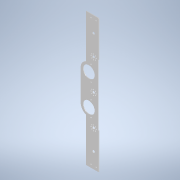
# Autodesk Inventor part: plate1
Saved by Autodesk Inventor 2020.1 (Build 241239000, 239)
## iProperties
Created: 2019-12-06
Part Number: plate1
Material: Aluminum 6061
Document SubType Name: Modeling
Designer: tbloo
Density: 2.7 g/cm^3
Appearance: Aluminum - Dark
Author: tbloo
Autodesk Inventor part; units mm, degrees
ref_plane "YZ Plane" through (0, 0, 0) normal (1, 0, 0) x (0, 1, 0)
ref_plane "XZ Plane" through (0, 0, 0) normal (0, 1, 0) x (-1, 0, 0)
ref_plane "XY Plane" through (0, 0, 0) normal (0, 0, 1) x (1, 0, 0)
sketch "Sketch1" plane through (0, 0, 0) normal (0, 0, 1) x (1, 0, 0)
  line L0 (48, -210) -> (48, -398)
  arc A0 (46, -400) -> (48, -398) centre (46, -398) ccw
  line L1 (46, -400) -> (-14, -400)
  line L2 (-16, -398) -> (-16, -210)
  arc A1 (-16, -398) -> (-14, -400) centre (-14, -398) ccw
  line L3 (48, -114.5) -> (48, -269.5)
  line L4 (48, 14) -> (48, -174)
  line L5 (-16, -174) -> (-16, 14)
  line L6 (-14, 16) -> (46, 16)
  arc A2 (-14, 16) -> (-16, 14) centre (-14, 14) ccw
  arc A3 (48, 14) -> (46, 16) centre (46, 14) ccw
  circle A4 centre (32, -184) radius 1.85
  circle A5 centre (37.6569, -186.3431) radius 1.85
  circle A6 centre (40, -192) radius 1.85
  circle A7 centre (32, -192) radius 4
  circle A8 centre (37.6569, -197.6569) radius 1.85
  circle A9 centre (24, -192) radius 1.85
  circle A10 centre (26.3431, -186.3431) radius 1.85
  circle A11 centre (26.3431, -197.6569) radius 1.85
  circle A12 centre (32, -200) radius 1.85
  circle A13 centre (37.6569, -101.6569) radius 1.85
  circle A14 centre (40, -96) radius 1.85
  circle A15 centre (37.6569, -90.3431) radius 1.85
  circle A16 centre (32, -88) radius 1.85
  circle A17 centre (32, -96) radius 4
  circle A18 centre (26.3431, -90.3431) radius 1.85
  circle A19 centre (24, -96) radius 1.85
  circle A20 centre (26.3431, -101.6569) radius 1.85
  circle A21 centre (32, -104) radius 1.85
  circle A22 centre (24, -288.0038) radius 1.85
  circle A23 centre (26.3431, -293.6606) radius 1.85
  circle A24 centre (32, -296.0038) radius 1.85
  circle A25 centre (37.6569, -293.6606) radius 1.85
  circle A26 centre (40, -288.0038) radius 1.85
  circle A27 centre (37.6569, -282.3469) radius 1.85
  circle A28 centre (32, -280.0038) radius 1.85
  circle A29 centre (26.3431, -282.3469) radius 1.85
  circle A30 centre (32, -288.0038) radius 4
  circle A31 centre (24, -264) radius 1.85
  circle A32 centre (24, -216) radius 1.85
  circle A33 centre (24, -168) radius 1.85
  circle A34 centre (24, -120) radius 1.85
  line L7 (-16, -210) -> (-16, -174)
  circle A35 centre (32, -352) radius 3.925
  circle A36 centre (32, -32) radius 3.925
  point P0 (0, 0)
  point P1 (16, -176)
  point P2 (16, -208)
  constraints: 37 centre point, 16 end point, 8 point on circle, 1 vertical, 12 other
extrude "Extrusion1" add sketch "Sketch1" along normal blind 2
sketch "Sketch3" plane through (0, 0, 2) normal (0, 0, 1) x (1, 0, 0)
  arc A0 (17, -162.5) -> (17, -125.5) centre (17, -144) ccw projected
  arc A1 (17, -258.5) -> (17, -221.5) centre (17, -240) ccw projected
  circle A2 centre (17, -144) radius 18.5
  circle A3 centre (17, -240) radius 18.5
  point P0 (0, 0)
  point P1 (17, -221.5)
  point P2 (17, -125.5)
  constraints: 2 centre point, 2 coincident, 1 concentric
extrude "Extrusion3" cut sketch "Sketch3" against normal through all
sketch "Sketch4" plane through (0, 0, 2) normal (0, 0, 1) x (1, 0, 0)
  circle A0 centre (17, -144) radius 18.65
  circle A1 centre (17, -240) radius 18.65
  arc A2 (8, -120.2479) -> (-8.4, -144) centre (17, -144) ccw
  arc A3 (-8.4, -240) -> (8, -263.7521) centre (17, -240) ccw
  line L0 (8, -263.7521) -> (8, -400)
  line L1 (8, 16) -> (8, -120.2479)
  line L2 (8, -400) -> (-14, -400)
  line L3 (8, 16) -> (-14, 16)
  arc A4 (-14, 16) -> (-16, 14) centre (-14, 14) ccw projected
  arc A5 (-16, -398) -> (-14, -400) centre (-14, -398) ccw projected
  line L4 (-8.4, -240) -> (-8.4, -208)
  line L5 (-8.4, -176) -> (-8.4, -144)
  line L6 (-16, 14) -> (-16, -398) projected
  line L7 (-16, -398) -> (-16, 14)
  line L8 (-8.4, -208) -> (-8.4, -176)
  point P0 (0, 0)
  dimension "d8" = 50.8
  constraints: 16 end point, 4 centre point, 4 point on circle, 3 vertical, 2 coincident, 1 collinear, 1 horizontal, 4 other
  measures "d8" diameter of A2
extrude "Extrusion4" cut sketch "Sketch4" against normal through all contours A2 L5 L8 L4 A3 L0 L2 A5 L6 A4 L3 L1
sketch "Sketch5" plane through (0, 0, 0) normal (0, 0, -1) x (-1, 0, 0)
  line L0 (-48, -96) -> (-46, -96)
  line L1 (-46, -288) -> (-48, -288)
  line L2 (-46, -288) -> (-46, -96)
  line L3 (-48, -398) -> (-48, 14) projected
  line L4 (-48, -96) -> (-48, -288)
  point P0 (0, 0)
  constraints: 8 end point, 2 horizontal, 1 collinear, 1 parallel, 4 other
extrude "Extrusion5" cut sketch "Sketch5" against normal through all
sketch "Sketch6" plane through (0, 0, 2) normal (0, 0, 1) x (1, 0, 0)
  circle A0 centre (40, 6.4) radius 1.85
  circle A1 centre (24, 6.4) radius 1.85
  circle A2 centre (40, -390.4) radius 1.85
  circle A3 centre (24, -390.4) radius 1.85
  point P0 (0, 0)
  constraints: 4 centre point, 8 other
extrude "Extrusion6" cut sketch "Sketch6" against normal through all
body "Solid1"
